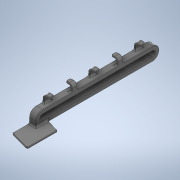
# Autodesk Inventor part: LED Arm
Saved by Autodesk Inventor 2020 (Build 240168000, 168)
## iProperties
Created: 2020-01-24
Part Number: LED Arm
Material: ABS Plastic
Document SubType Name: Modeling
Designer: Ishaan
Density: 1.06 g/cm^3
Appearance: Smooth - Black
Author: Ishaan
Autodesk Inventor part; units mm, degrees
ref_plane "YZ Plane" through (0, 0, 0) normal (1, 0, 0) x (0, 1, 0)
ref_plane "XZ Plane" through (0, 0, 0) normal (0, 1, 0) x (-1, 0, 0)
ref_plane "XY Plane" through (0, 0, 0) normal (0, 0, 1) x (1, 0, 0)
sketch "Sketch1" plane through (0, 0, 0) normal (0, 0, 1) x (1, 0, 0)
  line L0 (32.5, 0) -> (-32.5, 0) construction
  line L1 (32.5, 4) -> (-32.5, 4)
  line L2 (-32.5, -4) -> (32.5, -4)
  arc A0 (32.5, -4) -> (32.5, 4) centre (32.5, 0) ccw
  arc A1 (-32.5, 4) -> (-32.5, -4) centre (-32.5, 0) ccw
  line L3 (-32.5, 1.6) -> (32.5, 1.6)
  arc A2 (32.5, -1.6) -> (32.5, 1.6) centre (32.5, 0) ccw
  line L4 (32.5, -1.6) -> (-32.5, -1.6)
  arc A3 (-32.5, 1.6) -> (-32.5, -1.6) centre (-32.5, 0) ccw
  line L5 (-36.5, 0) -> (-36.5, -4)
  line L6 (-36.5, -4) -> (-32.5, -4)
  point P0 (0, 0)
  dimension "d0" = 8
  dimension "d1" = 65
  dimension "d2" = 3.2
  constraints: 16 end point, 9 point on circle, 5 tangent, 4 centre point, 2 parallel, 1 collinear, 1 horizontal, 1 midpoint, 3 other
  measures "d0" distance between parallel lines of L2 L1
  measures "d1" distance of L0.start L0.end
  measures "d2" distance between parallel lines of L4 L3
extrude "Extrusion1" add sketch "Sketch1" along normal mid plane 4
sketch "Sketch2" plane through (-36.5, -4, 2) normal (0, -1, 0) x (1, 0, 0)
  line L0 (69, -4) -> (0, -4) projected
  line L1 (0, -4) -> (-10, -4)
  line L2 (-10, -4) -> (-13.2154, 8)
  line L3 (-13.2154, 8) -> (4.7846, 8)
  line L4 (4.7846, 8) -> (6.9282, 0)
  line L5 (0, 0) -> (69, 0) projected
  line L6 (0, -4) -> (0, 0)
  line L7 (6.9282, 0) -> (0, 0)
  point P0 (36.5, -2)
  dimension "d5" = 18
  dimension "d6" = 10
  dimension "d7" = 105
  dimension "d9" = 8
  constraints: 12 end point, 2 parallel, 1 collinear, 1 horizontal, 1 perpendicular, 1 point on line
  measures "d5" distance of L2.end L3.end
  measures "d6" distance of L0.end L1.end
  measures "d7" angle of L1 L2
  measures "d9" distance between parallel lines of L5 L3
extrude "Extrusion2" add sketch "Sketch2" against normal blind 1
sketch "Sketch4" plane through (-32.5, 4, 2) normal (0, 1, 0) x (1, 0, 0)
  line L0 (0, 4) -> (0, 0) projected
  line L1 (65, 0) -> (0, 0) projected
  line L2 (65, 4) -> (65, 0) projected
  line L3 (0, 4) -> (65, 4) projected
  line L4 (4, 4) -> (7, 4)
  line L5 (7, 4) -> (7, 3)
  line L6 (7, 3) -> (4, 3)
  line L7 (4, 3) -> (4, 4)
  line L8 (4, 4) -> (7, 3) construction
  line L9 (7, 4) -> (4, 3) construction
  line L10 (17.5, 1) -> (20.5, 1)
  line L11 (20.5, 1) -> (20.5, 0)
  line L12 (20.5, 0) -> (17.5, 0)
  line L13 (17.5, 0) -> (17.5, 1)
  line L14 (17.5, 1) -> (20.5, 0) construction
  line L15 (20.5, 1) -> (17.5, 0) construction
  line L16 (44.5, 1) -> (47.5, 1)
  line L17 (47.5, 1) -> (47.5, 0)
  line L18 (47.5, 0) -> (44.5, 0)
  line L19 (44.5, 0) -> (44.5, 1)
  line L20 (44.5, 1) -> (47.5, 0) construction
  line L21 (47.5, 1) -> (44.5, 0) construction
  line L22 (65, 0) -> (0, 0) projected
  line L23 (0, 4) -> (65, 4) projected
  line L24 (34, 3) -> (31, 3)
  line L25 (31, 3) -> (31, 4)
  line L26 (31, 4) -> (34, 4)
  line L27 (34, 4) -> (34, 3)
  line L28 (34, 3) -> (31, 4) construction
  line L29 (31, 3) -> (34, 4) construction
  line L30 (61, 3) -> (58, 3)
  line L31 (58, 3) -> (58, 4)
  line L32 (58, 4) -> (61, 4)
  line L33 (61, 4) -> (61, 3)
  line L34 (61, 3) -> (58, 4) construction
  line L35 (58, 3) -> (61, 4) construction
  point P0 (32.5, 2)
  point P1 (5.5, 3.5)
  point P2 (19, 0.5)
  point P3 (46, 0.5)
  point P4 (32.5, 3.5)
  point P5 (59.5, 3.5)
  point P6 (32.5, 3.5)
  point P7 (17.5, 0)
  point P8 (20.5, 0)
  point P9 (7, 4)
  point P10 (4, 4)
  dimension "d25" = 3
  dimension "d26" = 1
  dimension "d27" = 13.5
  dimension "d28" = 13.5
  dimension "d29" = 13.5
  dimension "d30" = 13.5
  constraints: 60 end point, 18 parallel, 11 midpoint, 5 collinear, 5 horizontal, 5 perpendicular, 1 vertical alignment
  measures "d25" distance of L4.start L4.end
  measures "d26" distance of L4.end L5.end
  measures "d27" horizontal distance of point (19, 0.5) point (5.5, 3.5)
  measures "d28" horizontal distance of point (32.5, 3.5) point (19, 0.5)
  measures "d29" horizontal distance of point (46, 0.5) point (32.5, 3.5)
  measures "d30" horizontal distance of point (59.5, 3.5) point (46, 0.5)
extrude "Extrusion3" add sketch "Sketch4" along normal blind 4 contours L3 L5 L6 L7 | L13 L10 L11 L1 | L3 L27 L24 L25 | L19 L16 L17 L1 | L3 L33 L30 L31
sketch "Sketch5" plane through (-32.5, 8, 2) normal (0, 1, 0) x (1, 0, 0)
  line L0 (7, 4) -> (4, 4) projected
  line L1 (4, 4) -> (4, 3) projected
  line L2 (4, 3) -> (7, 3) projected
  line L3 (7, 3) -> (7, 4) projected
  line L4 (17.5, 1) -> (17.5, 0) projected
  line L5 (17.5, 0) -> (20.5, 0) projected
  line L6 (20.5, 0) -> (20.5, 1) projected
  line L7 (20.5, 1) -> (17.5, 1) projected
  line L8 (7, 4) -> (4, 4)
  line L9 (4, 4) -> (4, 0)
  line L10 (4, 0) -> (7, 0)
  line L11 (7, 0) -> (7, 4)
  line L12 (17.5, 0) -> (0, 0) projected
  line L13 (4, 4) -> (4, 3) projected
  point P0 (32.5, 2)
  dimension "d33" = 13.5
  constraints: 8 end point, 2 collinear, 2 parallel, 1 horizontal, 1 perpendicular
  measures "d33" distance between parallel lines of L1 L4
extrude "Extrusion4" add sketch "Sketch5" against normal blind 1 contours L3 L2 L1 L0 | L11 L10 L9 L2
pattern_linear "Rectangular Pattern1" count 5 spacing 13.5 along (1, 0, 0) of "Extrusion4"
fillet "Fillet4" radius 1 25 edges at (25.5, 7.5, 2) (28.5, 7.5, 2) (25.5, 4, -1.5) (28.5, 4, -1.5) (27, 4, -1) (13.5, 4, 1) (12, 4, 1.5) (15, 4, 1.5) (15, 7.5, -2) (12, 7.5, -2) (1.5, 7.5, 2) (-1.5, 7.5, 2) (1.5, 4, -1.5) (0, 4, -1) (-1.5, 4, -1.5) (-12, 4, 1.5) (-13.5, 4, 1) (-15, 4, 1.5) (-15, 7.5, -2) (-12, 7.5, -2) (-25.5, 4, -1.5) (-28.5, 4, -1.5) (-27, 4, -1) (-28.5, 7.5, 2) (-25.5, 7.5, 2)
fillet "Fillet5" radius 2 5 edges at (27, 8, -2) (13.5, 8, 2) (0, 8, -2) (-13.5, 8, 2) (-27, 8, -2)
fillet "Fillet6" radius 1 5 edges at (27, 7, -1) (13.5, 7, 1) (0, 7, -1) (-13.5, 7, 1) (-27, 7, -1)
fillet "Fillet1" radius 1 6 edges at (-49.7154, -3.5, 10) (-31.7154, -3.5, 10) (-29.5718, -3.5, 2) (-46.5, -3.5, -2) (-36.5, -3, 0) (-33.0359, -3, 2)
fillet "Fillet2" radius 0.25 91 edges at (-29.8048, -2.9914, 2.8695) (-29.4132, -2.6088, 2.2066) (-31.874, -3, 9.7934) (-40.4474, -3, 10) (-49.2055, -3, 9.6088) (-48.0383, -3, 3.7412) (-46.3414, -3, -1.7934) (-41.6163, -3, -2) (-36.7929, -2.7071, -2) (-36.5, -1, -2) (-35.3284, 2.8284, -2) (-31, 4, -2) (-13.5, 4, -2) (13.5, 4, -2) (31, 4, -2) (36.5, 0, -2) (-6.6163, -4, -2) (-46.3414, -4, -1.7934) (-48.0383, -4, 3.7412) (-49.2055, -4, 9.6088) (-40.4474, -4, 10) (-31.874, -4, 9.7934) (-30.6436, -4, 6) (-29.4132, -4, 2.2066) (1.8478, -4, 2) (36.5, 0, 2) (24.25, 4, 2) (0, 4, 2) (-24.25, 4, 2) (-35.3284, 2.8284, 2) (-36.5, -1, 2) (-36.7929, -2.7071, 2.2929) (-30.6783, -3, 6.1294) (-34.1, 0, -2) (0, -1.6, -2) (34.1, 0, -2) (0, 1.6, -2) (0, 1.6, 2) (34.1, 0, 2) (0, -1.6, 2) (-34.1, 0, 2) (-28.5, 6.7071, -0.7071) (-28.5, 7, 0.5) (-28.2071, 7, 1.7071) (-27, 7, 2) (-25.7929, 7, 1.7071) (-25.5, 7, 0.5) (-25.5, 6.7071, -0.7071) (-25.5, 5.5, -1) (-25.2071, 4.2929, -0.7071) (-28.7929, 4.2929, -0.7071) (-28.5, 5.5, -1) (-15, 5.5, 1) (-15, 6.7071, 0.7071) (-1.5, 7, 0.5) (-14.7071, 7, -1.7071) (-13.5, 7, -2) (-12.2929, 7, -1.7071) (1.5, 7, 0.5) (-12, 6.7071, 0.7071) (-12, 5.5, 1) (-11.7071, 4.2929, 0.7071) (-15.2929, 4.2929, 0.7071) (-1.5, 5.5, -1) (-1.5, 6.7071, -0.7071) (25.5, 7, 0.5) (-1.2071, 7, 1.7071) (27, 7, 2) (1.2071, 7, 1.7071) (28.5, 7, 0.5) (1.5, 6.7071, -0.7071) (1.5, 5.5, -1) (1.7929, 4.2929, -0.7071) (-1.7929, 4.2929, -0.7071) (12, 6.7071, 0.7071) (12.2929, 7, -1.7071) (13.5, 7, -2) (14.7071, 7, -1.7071) (15, 6.7071, 0.7071) (15, 5.5, 1) (15.2929, 4.2929, 0.7071) (11.7071, 4.2929, 0.7071) (12, 5.5, 1) (25.5, 5.5, -1) (25.2071, 4.2929, -0.7071) (25.7929, 7, 1.7071) (28.2071, 7, 1.7071) (28.5, 6.7071, -0.7071) (28.5, 5.5, -1) (28.7929, 4.2929, -0.7071) (25.5, 6.7071, -0.7071)
equation "\"d28\" = d27"
equation "\"d29\" = d28"
equation "\"d30\" = d29"
equation "\"d38\" = d33"
body "Solid1"
